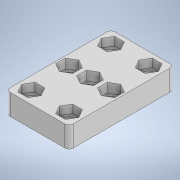
# Autodesk Inventor part: ViseA
Saved by Autodesk Inventor 2022 (Build 260153000, 153)
## iProperties
Created: 2021-11-10
Part Number: ViseA
Material: Genérico
Document SubType Name: Modeling
Designer: JK
Density: 1 g/cm^3
Appearance: Valor por defecto
Author: JK
Autodesk Inventor part; units mm, degrees
ref_plane "YZ Plane" through (0, 0, 0) normal (1, 0, 0) x (0, 1, 0)
ref_plane "XZ Plane" through (0, 0, 0) normal (0, 1, 0) x (-1, 0, 0)
ref_plane "XY Plane" through (0, 0, 0) normal (0, 0, 1) x (1, 0, 0)
sketch "Boceto1" plane through (0, 0, 0) normal (0, 1, 0) x (-1, 0, 0)
  line L0 (-15, 25) -> (15, 25)
  line L1 (15, 25) -> (15, -25)
  line L2 (15, -25) -> (-15, -25)
  line L3 (-15, -25) -> (-15, 25)
  line L4 (-15, 25) -> (15, -25) construction
  line L5 (15, 25) -> (-15, -25) construction
  point P0 (0, 0)
  dimension "d0" = 30
  dimension "d1" = 50
  constraints: 12 end point, 2 midpoint, 2 parallel, 1 horizontal, 1 perpendicular
  measures "d0" distance between parallel lines of L3 L1
  measures "d1" distance of L0.end L1.end
extrude "Extrusión1" add sketch "Boceto1" along normal blind 10
fillet "Empalme1" radius 2 4 edges at (-15, 5, -25) (-15, 5, 25) (15, 5, -25) (15, 5, 25)
sketch "Boceto2" plane through (0, 10, 0) normal (0, 1, 0) x (1, 0, 0)
  circle A0 centre (-10, 0) radius 2.7
  circle A1 centre (0, 0) radius 2.7
  circle A2 centre (10, 0) radius 2.7
  dimension "d5" = 5.4
  dimension "d6" = 10
  dimension "d7" = 10
  constraints: 3 centre point, 2 equal radius, 1 coincident
  measures "d5" diameter of A0
  measures "d6" distance of A0.centre point (0, 0)
  measures "d7" distance of point (0, 0) A2.centre
extrude "Extrusión2" cut sketch "Boceto2" against normal through all
sketch "Boceto3" plane through (0, 10, 0) normal (0, 1, 0) x (1, 0, 0)
  circle A0 centre (-9, -19) radius 2.7
  circle A1 centre (9, -19) radius 2.7
  circle A2 centre (-9, 19) radius 2.7
  circle A3 centre (9, 19) radius 2.7
  line L0 (-13, -25) -> (13, -25) projected
  line L1 (-15, 23) -> (-15, -23) projected
  line L2 (15, -23) -> (15, 23) projected
  line L3 (13, 25) -> (-13, 25) projected
  point P0 (0, 0)
  dimension "d10" = 5.4
  dimension "d11" = 6
  dimension "d12" = 6
  dimension "d13" = 6
  dimension "d14" = 6
  constraints: 4 centre point, 3 equal radius, 2 horizontal alignment, 2 vertical alignment
  measures "d10" diameter of A0
  measures "d11" distance from line of A0.centre L0
  measures "d12" distance from line of L1 A0.centre
  measures "d13" distance from line of L2 A1.centre
  measures "d14" distance from line of L3 A2.centre
extrude "Extrusión3" cut sketch "Boceto3" against normal through all
sketch "Boceto4" plane through (0, 10, 0) normal (0, 1, 0) x (1, 0, 0)
  circle A0 centre (-10, 0) radius 2.7 projected
  circle A1 centre (-10, 0) radius 4.05
  circle A2 centre (0, 0) radius 2.7 projected
  circle A3 centre (0, 0) radius 4.05
  circle A4 centre (10, 0) radius 2.7 projected
  circle A5 centre (10, 0) radius 4.05
  line L0 (-10, 4.6765) -> (-5.95, 2.3383)
  line L1 (-5.95, 2.3383) -> (-5.95, -2.3383)
  line L2 (-5.95, -2.3383) -> (-10, -4.6765)
  line L3 (-10, -4.6765) -> (-14.05, -2.3383)
  line L4 (-14.05, -2.3383) -> (-14.05, 2.3383)
  line L5 (-14.05, 2.3383) -> (-10, 4.6765)
  line L6 (0, 4.6765) -> (4.05, 2.3383)
  line L7 (4.05, 2.3383) -> (4.05, -2.3383)
  line L8 (4.05, -2.3383) -> (0, -4.6765)
  line L9 (0, -4.6765) -> (-4.05, -2.3383)
  line L10 (-4.05, -2.3383) -> (-4.05, 2.3383)
  line L11 (-4.05, 2.3383) -> (0, 4.6765)
  line L12 (10, 4.6765) -> (14.05, 2.3383)
  line L13 (14.05, 2.3383) -> (14.05, -2.3383)
  line L14 (14.05, -2.3383) -> (10, -4.6765)
  line L15 (10, -4.6765) -> (5.95, -2.3383)
  line L16 (5.95, -2.3383) -> (5.95, 2.3383)
  line L17 (5.95, 2.3383) -> (10, 4.6765)
  dimension "d17" = 8.1
  constraints: 36 end point, 6 coincident, 3 centre point, 3 tangent, 3 vertical, 2 equal radius, 39 other
  measures "d17" diameter of A1
extrude "Extrusión4" cut sketch "Boceto4" against normal blind 4.5 contours A0 | A1 | L1 L2 A1 | A1 L0 L1 | A1 L5 L0 | L2 L3 A1 | A1 L4 L5 | L3 L4 A1 | A2 | A3 | L7 L8 A3 | A3 L6 L7 | A3 L11 L6 | L8 L9 A3 | A3 L10 L11 | L9 L10 A3 | A4 | A5 | L13 L14 A5 | A5 L12 L13 | A5 L17 L12 | L14 L15 A5 | A5 L16 L17 | L15 L16 A5
sketch "Boceto5" plane through (0, 10, 0) normal (0, 1, 0) x (1, 0, 0)
  circle A0 centre (-9, -19) radius 2.7 projected
  circle A1 centre (-9, -19) radius 4.05
  line L0 (-13.6765, -18.9802) -> (-11.3211, -14.9401)
  line L1 (-11.3211, -14.9401) -> (-6.6446, -14.96)
  line L2 (-6.6446, -14.96) -> (-4.3235, -19.0198)
  line L3 (-4.3235, -19.0198) -> (-6.6789, -23.0599)
  line L4 (-6.6789, -23.0599) -> (-11.3554, -23.04)
  line L5 (-11.3554, -23.04) -> (-13.6765, -18.9802)
  point P0 (0, 0)
  dimension "d20" = 8.1
  constraints: 12 end point, 2 coincident, 1 centre point, 1 tangent, 13 other
  measures "d20" diameter of A1
extrude "Extrusión5" cut sketch "Boceto5" against normal blind 4 contours A0 | A1 | A1 L2 L3 | A1 L1 L2 | L3 L4 A1 | A1 L0 L1 | L4 L5 A1 | A1 L5 L0
pattern_linear "Patrón rectangular1" count 2 spacing 38 along (0, 0, -1) count 2 spacing 18 along (1, 0, 0) of "Extrusión5"
